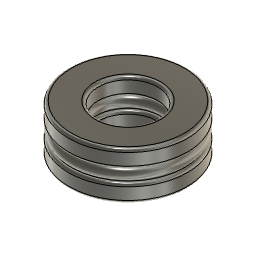
final_assembly (Autodesk Fusion 360 archive; units mm, degrees)
design "F5-10M Thrust Bearing"
Autodesk Fusion 360 part; units mm, degrees
sketch "Sketch1" plane through (0, 0, 0) normal (0, 0, 1) x (1, 0, 0)
  circle A0 centre (0, 0) radius 5
  circle A1 centre (0, 0) radius 2.5
  dimension "d1" = 10
  dimension "d2" = 5
  constraint coincident A0.centre A1.centre
  measures "d1" diameter of A0
  measures "d2" diameter of A1
extrude "Extrude1" add sketch "Sketch1" along normal blind 1.5 makes body 1
extrude "Extrude2" add 1 faces at (4.1387, -0.3726, 1.5) along direction (0, 0, 1) blind 1 separate body on bodies 1 makes body 2
extrude "Extrude3" add 1 faces at (4.1387, -0.3726, 2.5) along direction (0, 0, 1) blind 1.5 separate body on bodies 2 makes body 3
copy_body "Body->Comp1" bodies 1 removing the originals makes body 4 in component "Base"
copy_body "Body->Comp2" bodies 2 removing the originals makes body 5 in component "Middle"
copy_body "Body->Comp3" bodies 3 removing the originals makes body 6 in component "Top"
fillet "Fillet1" radius 0.5 4 edges at (-4.6616, -1.8081, 2.5) (-4.6616, -1.8081, 1.5) (-2.3308, 0.904, 2.5) (-2.3308, 0.904, 1.5) on bodies 5 in component "Middle"
fillet "Fillet1'" radius 0.25 3 edges at (-4.6616, -1.8081, 1.5) (-4.6616, -1.8081, 0) (-2.3308, 0.904, 1.5) on bodies 4 in component "Base"
fillet "Fillet1''" radius 0.25 4 edges at (-4.6616, -1.8081, 2.5) (-4.6616, -1.8081, 4) (-2.3308, 0.904, 4) (-2.3308, 0.904, 2.5) on bodies 6 in component "Top"
component "Base" placed x (1, 0, 0) y (0, 1, 0) z (0, 0, 1) at (0, 0, 0)
component "Middle" placed x (1, 0, 0) y (0, 1, 0) z (0, 0, 1) at (0, 0, 0)
component "Top" placed x (0, -1, 0) y (1, 0, 0) z (0, 0, 1) at (0, 0, 0)

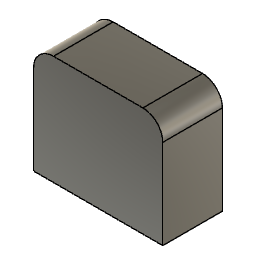
design "cover motor top"
Autodesk Fusion 360 part; units mm, degrees
sketch "Sketch1" plane through (0, 0, 0) normal (0, 1, 0) x (1, 0, 0)
  line L0 (25.6354, -40) -> (70.6354, -40)
  line L1 (80.6354, -30) -> (80.6354, 15)
  line L2 (80.6354, 15) -> (15.6354, 15)
  line L3 (15.6354, 15) -> (15.6354, -30)
  arc A0 (15.6354, -30) -> (25.6354, -40) centre (25.6354, -30) ccw
  arc A1 (70.6354, -40) -> (80.6354, -30) centre (70.6354, -30) ccw
  dimension "d1" = 65
  dimension "d2" = 55
  dimension "d3" = 10
  dimension "d4" = 10
  constraint horizontal L0
  constraint vertical L1
  constraint horizontal L2
  constraint vertical L3
  constraint tangent L0 A0
  constraint tangent L3 A0
  constraint tangent L0 A1
  constraint tangent L1 A1
  measures "d1" distance of L1 L3
  measures "d2" distance of L0 L2
  measures "d3" radius of A0
  measures "d4" radius of A1
extrude "Extrude2" add sketch "Sketch1" along normal blind 30
shell "Shell2" thickness 3 removed faces 1 at (58.9688, 20, -15)
sketch "Sketch2" plane through (0, 0, 0) normal (1, 0, 0) x (0, 1, 0)
  line L0 (21, 15.6496) -> (10, 15.6496)
  line L1 (10, 15.6496) -> (10, -16.8071)
  line L2 (10, -16.8071) -> (21, -16.8071)
  line L3 (21, -16.8071) -> (21, 15.6496)
  dimension "d11" = 11
  constraint horizontal L0
  constraint vertical L1
  constraint horizontal L2
  constraint vertical L3
  measures "d11" distance of L1 L3
extrude "Extrude3" cut sketch "Sketch2" along normal blind 25

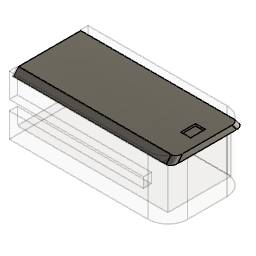
design "box cover boards"
Autodesk Fusion 360 part; units mm, degrees
sketch "Sketch1" plane through (0, 0, 0) normal (0, 1, 0) x (1, 0, 0) in component "box"
  line L0 (-11, -75) -> (150, -75)
  line L1 (150, -75) -> (150, -15)
  line L2 (150, -15) -> (-11, -15)
  line L3 (-11, -15) -> (-11, -75)
  dimension "d1_1" = 60
  dimension "d2_1" = 161
  constraint horizontal L0
  constraint vertical L1
  constraint horizontal L2
  constraint vertical L3
  measures "d1_1" distance of L0 L2
  measures "d2_1" distance of L1 L3
extrude "Extrude1" add sketch "Sketch1" along normal blind 80 makes body 1 in component "box"
shell "Shell1" thickness 8 removed faces 2 at (42.6667, 53.3333, 75) at (-11, 26.6667, 35) on bodies 1 in component "box"
sketch "Sketch3" plane through (150, 0, 0) normal (1, 0, 0) x (0, 1, 0) in component "box"
  line L0 (0, 75) -> (0, 15)
  line L1 (0, 15) -> (80, 15)
  line L2 (80, 15) -> (80, 75)
  line L3 (80, 75) -> (0, 75)
  line L4 (8, 75) -> (2.9447, 68.7997)
  line L5 (40, 75) -> (40, 68.7997) construction
  line L6 (40, 68.7997) -> (2.9447, 68.7997)
  line L7 (72, 75) -> (77.0553, 68.7997)
  line L8 (40, 68.7997) -> (77.0553, 68.7997)
  point P0 (8, 75)
  point P1 (72, 75)
  dimension "d13_1" = 8
  constraint coincident P0 L4.start
  constraint midpoint L3 L5.start
  constraint perpendicular L3 L5
  constraint horizontal L4.end L5.end
  constraint symmetric P0 L5 P1
  constraint symmetric L4.end L5 L7.end
  constraint symmetric L6.start L5 L8.start
  measures "d13_1" distance of P0 L4.end
extrude "Extrude3" cut sketch "Sketch3" against normal blind 200 contours L3 L4 L6 L7 L8 bodies 1 in component "box"
fillet "Fillet3" radius 20 1 edges at (150, 0, 45) on bodies 1 in component "box"
fillet "Fillet4" radius 20 1 edges at (150, 80, 45) on bodies 1 in component "box"
sketch "Sketch1 (2)" plane through (-86.6627, 0, 0) normal (-1, 0, 0) x (0, -1, 0)
  line L0 (4.4676, 66.1951) -> (4.4676, 6.1951)
  line L1 (4.4676, 6.1951) -> (84.4676, 6.1951)
  line L2 (84.4676, 6.1951) -> (84.4676, 66.1951)
  line L3 (76.4676, 14.1951) -> (12.4676, 14.1951)
  line L4 (12.4676, 14.1951) -> (12.4676, 59.9948)
  circle A0 centre (80, -30) radius 1.5
  circle A1 centre (-120, -30) radius 1.5
  line L5 (81.5228, 59.9948) -> (76.4676, 59.9948)
  line L6 (7.4123, 59.9948) -> (12.4676, 66.1951)
  line L7 (12.4676, 66.1951) -> (4.4676, 66.1951)
  line L8 (76.4676, 59.9948) -> (76.4676, 14.1951)
  line L9 (84.4676, 66.1951) -> (76.4676, 66.1951)
  line L10 (76.4676, 66.1951) -> (81.5228, 59.9948)
  line L11 (12.4676, 59.9948) -> (7.4123, 59.9948)
  dimension "d1" = 3
  dimension "d2" = 3
  measures "d1" diameter of A0
  measures "d2" diameter of A1
sketch "Sketch2" plane through (0, -48.0314, 0) normal (0, -1, 0) x (1, 0, 0)
  line L0 (54.9401, 42.0285) -> (54.9401, 102.0285)
  line L1 (54.9401, 102.0285) -> (-86.0599, 102.0285)
  line L2 (-86.0599, 102.0285) -> (-86.0599, 42.0285)
  line L3 (-86.0599, 42.0285) -> (54.9401, 42.0285)
  line L4 (54.9401, 72.0285) -> (-86.0599, 72.0285) construction
  line L5 (50.1688, 72.0285) -> (50.1688, 67.0285)
  line L6 (50.1688, 72.0285) -> (50.1688, 77.0285)
  line L7 (50.1688, 77.0285) -> (-86.0599, 77.0285)
  line L8 (50.1688, 67.0285) -> (-86.0599, 67.0285)
  dimension "d5" = 5
  dimension "d6" = 5
  constraint midpoint L0 L4.start
  constraint midpoint L2 L4.end
  constraint coincident L4 L5.start
  constraint perpendicular L4 L5
  constraint perpendicular L4 L6
  constraint coincident L2 L7.end
  constraint perpendicular L2 L7
  constraint coincident L2 L8.end
  constraint perpendicular L2 L8
  measures "d5" distance of L5.start L5.end
  measures "d6" distance of L5.start L6.end
extrude "Extrude8" cut sketch "Sketch2" against normal blind 30 contours L2 L5 L6 L7 L8 sketch seen with x (1, 0, 0) y (0, 1, 0) z (0, 0, 1) at (75.0599, 48.0314, -27.0285) bodies 1 in component "box"
sketch "Sketch3 (2)" plane through (0, 31.9686, 0) normal (0, 1, 0) x (-1, 0, 0)
  line L0 (-54.9401, 102.0285) -> (-54.9401, 42.0285)
  line L1 (-54.9401, 42.0285) -> (86.0599, 42.0285)
  line L2 (86.0599, 42.0285) -> (86.0599, 102.0285)
  line L3 (86.0599, 102.0285) -> (-54.9401, 102.0285)
  line L4 (67.5, 90.4008) -> (86.0599, 90.4008)
  line L5 (86.0599, 90.4008) -> (86.0599, 77.7208)
  line L6 (86.0599, 77.7208) -> (67.5, 77.7208)
  line L7 (65, 80.2208) -> (65, 87.9008)
  arc A0 (67.5, 90.4008) -> (65, 87.9008) centre (67.5, 87.9008) ccw
  arc A1 (65, 80.2208) -> (67.5, 77.7208) centre (67.5, 80.2208) ccw
  dimension "d9" = 2.5
  constraint horizontal L4
  constraint vertical L5
  constraint horizontal L6
  constraint vertical L7
  constraint coincident L2 L5.end
  constraint tangent L4 A0
  constraint tangent L7 A0
  constraint tangent L6 A1
  constraint tangent L7 A1
  constraint equal A0 A1
  measures "d9" radius of A0
extrude "Extrude9" cut sketch "Sketch3 (2)" against normal blind 20 contours L2 L4 L5 L6 L7 A0 A1 sketch seen with x (1, 0, 0) y (0, 1, 0) z (0, 0, 1) at (75.0599, 48.0314, -27.0285) bodies 1 in component "box"
sketch "Sketch1 (3)" plane through (74.9401, 0, 0) normal (1, 0, 0) x (0, 1, 0) in component "lid"
  line L0 (11.9686, 42.0285) -> (11.9686, 95.8282)
  line L1 (11.9686, 95.8282) -> (-28.0314, 95.8282)
  line L2 (-28.0314, 95.8282) -> (-28.0314, 42.0285)
  line L3 (-28.0314, 42.0285) -> (11.9686, 42.0285)
  line L4 (-48.0314, 102.0285) -> (-40.0314, 102.0285)
  line L5 (-40.0314, 102.0285) -> (-45.0867, 95.8282)
  line L6 (-45.0867, 95.8282) -> (-28.0314, 95.8282)
  line L7 (11.9686, 95.8282) -> (-28.0314, 95.8282)
  line L8 (11.9686, 95.8282) -> (29.0239, 95.8282)
  line L9 (29.0239, 95.8282) -> (23.9686, 102.0285)
  line L10 (23.9686, 102.0285) -> (31.9686, 102.0285)
  line L11 (-48.0314, 102.2785) -> (-39.505, 102.2785)
  line L12 (-39.505, 102.2785) -> (-44.5603, 96.0782)
  line L13 (-44.5603, 96.0782) -> (-28.0314, 96.0782)
  line L14 (11.9686, 96.0782) -> (-28.0314, 96.0782)
  line L15 (11.9686, 96.0782) -> (28.4975, 96.0782)
  line L16 (28.4975, 96.0782) -> (23.4422, 102.2785)
  line L17 (23.4422, 102.2785) -> (31.9686, 102.2785)
  line L18 (23.4422, 102.2785) -> (-39.505, 102.2785)
  dimension "d12" = -0.25
  constraint parallel L11 L18
extrude "Extrude1'" add sketch "Sketch1 (3)" against normal blind 160 separate body contours L12 L13 L14 L15 L16 L18 makes body 2 in component "lid"
fillet "Fillet1" radius 5 1 edges at (74.9401, -42.0326, 99.1784) on bodies 2 in component "lid"
fillet "Fillet2" radius 5 1 edges at (74.9401, 25.9698, 99.1784) on bodies 2 in component "lid"
sketch "Sketch2 (2)" plane through (0, 0, 102.2785) normal (0, 0, 1) x (-1, 0, 0) in component "lid"
  ellipse E0 centre (-69.9401, -16.991) end of major axis (-69.9401, -23.4422) minor radius 5 (-74.9401, -16.991) -> (-69.9401, -23.4422) ccw
  line L0 (-69.9401, -23.4422) -> (85.0599, -23.4422)
  line L1 (85.0599, -23.4422) -> (85.0599, 39.505)
  line L2 (85.0599, 39.505) -> (-69.9401, 39.505)
  ellipse E1 centre (-69.9401, 33.0538) end of major axis (-69.9401, 39.505) minor radius 5 (-69.9401, 39.505) -> (-74.9401, 33.0538) ccw
  line L3 (-74.9401, 33.0538) -> (-74.9401, -16.991)
  line L4 (-65, 14.9834) -> (-55, 14.9834)
  line L5 (-55, 14.9834) -> (-55, 0.0818)
  line L6 (-55, 0.0818) -> (-65, 0.0818)
  line L7 (-65, 0.0818) -> (-65, 14.9834)
  constraint horizontal L4
  constraint vertical L5
  constraint horizontal L6
  constraint vertical L7
extrude "Extrude2" cut sketch "Sketch2 (2)" against normal blind 2 contours L4 L5 L6 L7 bodies 2 in component "lid"
component "box" placed x (1, 0, 0) y (0, 1, 0) z (0, 0, 1) at (-75.0599, -48.0314, 27.0285)
component "lid" placed x (1, 0, 0) y (0, 1, 0) z (0, 0, 1) at (0, 0, 0)

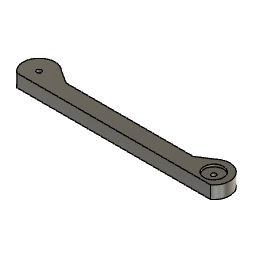
design "link 3"
Autodesk Fusion 360 part; units mm, degrees
sketch "Sketch2" plane through (0, 0, 0) normal (0, 0, 1) x (1, 0, 0)
  line L0 (91, -8) -> (-31, -8)
  line L1 (-10, 2.005) -> (70, 2.005)
  line L2 (70, 2.005) -> (77.9321, 7.0743)
  line L3 (-10, 2.005) -> (-17.9321, 7.0743)
  arc A0 (-17.9321, 7.0743) -> (-31, -8) centre (-25, 0) ccw
  arc A1 (91, -8) -> (77.9321, 7.0743) centre (85, 0) ccw
  dimension "d20" = 20
  dimension "d21" = 20
  dimension "d22" = 110
  dimension "d24" = 10.005
  constraint horizontal L0
  constraint parallel L0 L1
  measures "d20" diameter of A0
  measures "d21" diameter of A1
  measures "d22" distance of A0.centre A1.centre
  measures "d24" distance of L0 L1
extrude "Extrude1" add sketch "Sketch2" along normal blind 8
sketch "Sketch3" plane through (0, 0, 8) normal (0, 0, 1) x (-1, 0, 0)
  line L0 (10, -2.005) -> (17.9321, -7.0743)
  arc A0 (17.9321, -7.0743) -> (31, 8) centre (25, 0) ccw
  line L1 (31, 8) -> (-91, 8)
  arc A1 (-91, 8) -> (-77.9321, -7.0743) centre (-85, 0) ccw
  line L2 (-77.9321, -7.0743) -> (-70, -2.005)
  line L3 (-70, -2.005) -> (10, -2.005)
  circle A2 centre (-85, 0) radius 6.1
  dimension "d28" = 12.2
  constraint concentric A1 A2
  measures "d28" diameter of A2
sketch "Sketch4" plane through (0, 0, 0) normal (0, 0, -1) x (1, 0, 0)
  line L0 (-17.9321, -7.0743) -> (-10, -2.005)
  line L1 (-10, -2.005) -> (70, -2.005)
  line L2 (70, -2.005) -> (77.9321, -7.0743)
  arc A0 (77.9321, -7.0743) -> (91, 8) centre (85, 0) ccw
  line L3 (91, 8) -> (-31, 8)
  arc A1 (-31, 8) -> (-17.9321, -7.0743) centre (-25, 0) ccw
  circle A2 centre (-25, 0) radius 6.1
  dimension "d32" = 12.2
  constraint concentric A1 A2
  measures "d32" diameter of A2
extrude "Extrude4" cut sketch "Sketch4" against normal blind 1.5 contours A2
extrude "Extrude5" cut sketch "Sketch3" against normal blind 1.5 contours A2
sketch "Sketch5" plane through (0, 0, 0) normal (0, 0, -1) x (1, 0, 0)
  circle A0 centre (-25, 0) radius 6.1
  line L0 (-17.9321, -7.0743) -> (-10, -2.005)
  line L1 (-10, -2.005) -> (70, -2.005)
  line L2 (70, -2.005) -> (77.9321, -7.0743)
  arc A1 (77.9321, -7.0743) -> (91, 8) centre (85, 0) ccw
  line L3 (91, 8) -> (-31, 8)
  arc A2 (-31, 8) -> (-17.9321, -7.0743) centre (-25, 0) ccw
  circle A3 centre (85, 0) radius 1.5
  dimension "d39" = 3
  constraint concentric A1 A3
  measures "d39" diameter of A3
extrude "Extrude7" cut sketch "Sketch5" against normal blind 13 contours A3
sketch "Sketch6" plane through (0, 0, 8) normal (0, 0, 1) x (-1, 0, 0)
  circle A0 centre (-85, 0) radius 6.1
  line L0 (10, -2.005) -> (17.9321, -7.0743)
  arc A1 (17.9321, -7.0743) -> (31, 8) centre (25, 0) ccw
  line L1 (31, 8) -> (-91, 8)
  arc A2 (-91, 8) -> (-77.9321, -7.0743) centre (-85, 0) ccw
  line L2 (-77.9321, -7.0743) -> (-70, -2.005)
  line L3 (-70, -2.005) -> (10, -2.005)
  circle A3 centre (25, 0) radius 1.5
  dimension "d44" = 3
  constraint concentric A1 A3
  measures "d44" diameter of A3
extrude "Extrude8" cut sketch "Sketch6" against normal blind 11 contours A3
component "arm1" placed x (1, 0, 0) y (0, 1, 0) z (0, 0, 1) at (0, 0, 0)

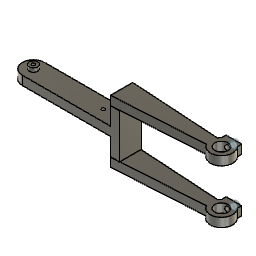
design "link 2 (EE)"
Autodesk Fusion 360 part; units mm, degrees
sketch "Sketch1" plane through (0, 0, 0) normal (0, 0, 1) x (1, 0, 0)
  circle A0 centre (-60, 0) radius 3.75 construction
  circle A1 centre (-60, 0) radius 10 construction
  line L0 (-120, 10) -> (-40.6913, 10)
  line L1 (-120, -10) -> (-40.6913, -10)
  line L2 (-40.6913, 10) -> (-40.6913, -10)
  arc A2 (-120, 10) -> (-120, -10) centre (-120, 0) ccw
  dimension "d1" = 20
  dimension "d2" = 7.5
  dimension "d3" = 60
  dimension "d4" = 20
  constraint concentric A0 A1
  constraint tangent L0 A2
  constraint horizontal L0
  constraint tangent L1 A2
  constraint parallel L0 L1
  constraint perpendicular L1 L2
  measures "d1" diameter of A2
  measures "d2" diameter of A0
  measures "d3" distance of A2.centre A0.centre
  measures "d4" diameter of A1
extrude "Extrude1" add sketch "Sketch1" along normal blind 8 makes body 1
sketch "Sketch2" plane through (0, 0, 0) normal (0, 1, 0) x (1, 0, 0)
  line L0 (-43, -20) -> (-35, -20)
  line L1 (-35, -20) -> (-35, 20)
  line L2 (-35, 20) -> (-43, 20)
  line L3 (-43, 20) -> (-43, -20)
  dimension "d7" = 8
  dimension "d8" = 40
  constraint horizontal L0
  constraint vertical L1
  constraint horizontal L2
  constraint vertical L3
  measures "d7" distance of L1 L3
  measures "d8" distance of L0 L2
extrude "Extrude2" add sketch "Sketch2" along normal blind 10 and the other way blind 10 separate body makes body 2
copy_body "Body->Comp1" bodies 1 removing the originals makes body 3 in component "section 1 (l4)"
copy_body "Body->Comp2" bodies 2 removing the originals makes body 4 in component "middle bit"
sketch "Sketch3" plane through (0, 0, 8) normal (0, 0, 1) x (-1, 0, 0)
  line L0 (40.6913, -10) -> (120, -10)
  arc A0 (120, -10) -> (120, 10) centre (120, 0) ccw
  line L1 (120, 10) -> (40.6913, 10)
  line L2 (40.6913, 10) -> (40.6913, -10)
  line L3 (25, -10) -> (25, 10)
  line L4 (25, -10) -> (-56.3022, -4.9345)
  line L5 (25, 10) -> (-56.3022, 4.9345)
  line L6 (-58, -11) -> (-72.0708, -11)
  line L7 (-72.0708, -11) -> (-72.0708, -7.0714)
  line L8 (-58, -7.0714) -> (-58, -11)
  arc A1 (-58, -7.1414) -> (-56.3022, -4.9345) centre (-65, 0) ccw
  arc A2 (-56.3022, 4.9345) -> (-72.0708, -7.0714) centre (-65, 0) ccw
  circle A3 centre (-65, 0) radius 6
  dimension "d17" = 20
  dimension "d18" = 90
  dimension "d19" = 12
  constraint vertical L3
  constraint coincident L5.end A1
  constraint horizontal L6
  constraint vertical L7
  constraint vertical L8
  constraint coincident L8 A1.start
  constraint concentric A1 A2
  constraint concentric A2 A3
  measures "d17" diameter of A1
  measures "d18" distance of A1.centre L3
  measures "d19" diameter of A3
extrude "Extrude3" add sketch "Sketch3" along normal blind 8 separate body contours L3 L4 L5 L6 L7 L8 A1 A2 makes body 5
sketch "Sketch5" plane through (0, 0, 0) normal (0, 0, 1) x (1, 0, 0)
  circle A0 centre (65.005, -0.1371) radius 6
  line L0 (-25, -10) -> (-25, 10)
  line L1 (-25, 10) -> (56.3881, 4.9373)
  line L2 (-25, -10) -> (56.247, -4.9638)
  line L3 (71.9058, 7.1002) -> (72, 7.1002)
  line L4 (72, 7.1002) -> (72, 11)
  line L5 (72, 11) -> (58.1042, 11)
  line L6 (58.1042, 11) -> (58.1042, 7.1002)
  arc A1 (56.247, -4.9638) -> (71.9058, 7.1002) centre (65.005, -0.1371) ccw
  arc A2 (58.1042, 7.1002) -> (56.3881, 4.9373) centre (65.005, -0.1371) ccw
  dimension "d24" = 20
  dimension "d25" = 12
  constraint concentric A0 A1
  constraint vertical L0
  constraint horizontal L3
  constraint vertical L4
  constraint horizontal L5
  constraint vertical L6
  constraint coincident L6.end A1
  constraint concentric A1 A2
  measures "d24" diameter of A1
  measures "d25" diameter of A0
extrude "Extrude4" add sketch "Sketch5" against normal blind 8 separate body makes body 6
copy_body "Body->Comp3" bodies 5 removing the originals makes body 7 in component "top arm "
copy_body "Body->Comp4" bodies 6 removing the originals makes body 8 in component "bottom arm"
cylinder "CylinderPrimitive1" add diameter 7.7 height 3.5 placed x (1, 0, 0) y (0, 1, 0) z (0, 0, 1) at (-120, 0, 8) bodies 3 in component "section 1 (l4)"
cylinder "CylinderPrimitive2" add diameter 7.7 height 3.5 placed x (0, 1, 0) y (1, 0, 0) z (0, 0, -1) at (-57.218, 0, 0) bodies 3 in component "section 1 (l4)"
sketch "Sketch9" plane through (-0.218, 11, 0) normal (0, 1, 0) x (-1, 0, 0)
  line L0 (-54.2887, 20) -> (-40.218, 20)
  line L1 (-40.218, 20) -> (-40.218, 28)
  line L2 (-40.218, 28) -> (-54.2887, 28)
  line L3 (-54.2887, 28) -> (-54.2887, 20)
  circle A0 centre (-47.1099, 23.7364) radius 2.5
  circle A1 centre (-47.2533, -23.9842) radius 2.5
  dimension "d44" = 5
  dimension "d45" = 5
  measures "d44" diameter of A0
  measures "d45" diameter of A1
extrude "Extrude1'" cut sketch "Sketch9" against normal blind 10 contours A0 | A1 sketch seen with x (1, 0, 0) y (0, 1, 0) z (0, 0, 1) at (18, 0, -12) bodies 7 in component "top arm "
extrude "Extrude1''" cut sketch "Sketch9" against normal blind 10 contours A0 | A1 sketch seen with x (1, 0, 0) y (0, 1, 0) z (0, 0, 1) at (18, 0, 20) bodies 8 in component "bottom arm"
combine "Combine1" operation add target body 3 tool bodies 7 8 4 body 7 seen with x (1, 0, 0) y (0, 1, 0) z (0, 0, 1) at (-15.6913, 0, 16) body 8 seen with x (1, 0, 0) y (0, 1, 0) z (0, 0, 1) at (-15.6913, 0, -16) body 4 seen with x (1, 0, 0) y (0, 1, 0) z (0, 0, 1) at (2.3087, 0, 4) in component "section 1 (l4)"
sketch "Sketch10" plane through (0, 0, 7.5) normal (0, 0, 1) x (-1, 0, 0)
  circle A0 centre (122.3087, 0) radius 3.85
  circle A1 centre (122.3087, 0) radius 1.5
  dimension "d50" = 3
  constraint concentric A0 A1
  measures "d50" diameter of A1
extrude "Extrude1'''" cut sketch "Sketch10" against normal blind 18 contours A1 sketch seen with x (1, 0, 0) y (0, 1, 0) z (0, 0, 1) at (2.3087, 0, 4) bodies 3 in component "section 1 (l4)"
sketch "Sketch11" plane through (0, 0, -7.5) normal (0, 0, -1) x (1, 0, 0)
  circle A0 centre (-59.5266, 0) radius 3.85
  circle A1 centre (-59.5266, 0) radius 1.5
  dimension "d53" = 3
  constraint concentric A0 A1
  measures "d53" diameter of A1
extrude "Extrude2'" cut sketch "Sketch11" against normal blind 14 contours A1 sketch seen with x (1, 0, 0) y (0, 1, 0) z (0, 0, 1) at (2.3087, 0, 4) bodies 3 in component "section 1 (l4)"
component "section 1 (l4)" placed x (1, 0, 0) y (0, 1, 0) z (0, 0, 1) at (-2.3087, 0, -4)
component "middle bit" placed x (1, 0, 0) y (0, 1, 0) z (0, 0, 1) at (0, 0, 0)
component "top arm " placed x (1, 0, 0) y (0, 1, 0) z (0, 0, 1) at (-18, 0, 12)
component "bottom arm" placed x (1, 0, 0) y (0, 1, 0) z (0, 0, 1) at (-18, 0, -20)
named bodies: "section 1 (l4)", "middle bit", "top arm", "bottom arm"

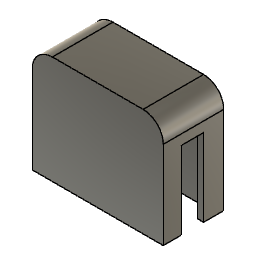
design "cover motor bottom"
Autodesk Fusion 360 part; units mm, degrees
sketch "Sketch1" plane through (0, 0, 0) normal (0, 1, 0) x (1, 0, 0)
  line L0 (25.6354, -40) -> (70.6354, -40)
  line L1 (80.6354, -30) -> (80.6354, 13.5)
  line L2 (80.6354, 13.5) -> (15.6354, 13.5)
  line L3 (15.6354, 13.5) -> (15.6354, -30)
  arc A0 (15.6354, -30) -> (25.6354, -40) centre (25.6354, -30) ccw
  arc A1 (70.6354, -40) -> (80.6354, -30) centre (70.6354, -30) ccw
  dimension "d1" = 65
  dimension "d2" = 53.5
  dimension "d3" = 10
  dimension "d4" = 10
  constraint horizontal L0
  constraint vertical L1
  constraint horizontal L2
  constraint vertical L3
  constraint tangent L0 A0
  constraint tangent L3 A0
  constraint tangent L0 A1
  constraint tangent L1 A1
  measures "d1" distance of L1 L3
  measures "d2" distance of L0 L2
  measures "d3" radius of A0
  measures "d4" radius of A1
extrude "Extrude2" add sketch "Sketch1" along normal blind 30
shell "Shell2" thickness 3 removed faces 1 at (58.9688, 20, -13.5)
sketch "Sketch3" plane through (80.6354, 0, 0) normal (1, 0, 0) x (0, 1, 0)
  line L0 (0, 30) -> (0, -13.5)
  line L1 (0, -13.5) -> (30, -13.5)
  line L2 (30, -13.5) -> (30, 30)
  line L3 (30, 30) -> (0, 30)
  line L4 (9, 25.0348) -> (20, 25.0348)
  line L5 (20, 25.0348) -> (20, -16.6958)
  line L6 (20, -16.6958) -> (9, -16.6958)
  line L7 (9, -16.6958) -> (9, 25.0348)
  dimension "d18" = 11
  constraint horizontal L4
  constraint vertical L5
  constraint horizontal L6
  constraint vertical L7
  measures "d18" distance of L5 L7
extrude "Extrude4" cut sketch "Sketch3" against normal blind 10 contours L1 L4 L5 L7 | L1 L5 L6 L7
